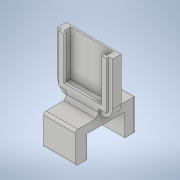
# Autodesk Inventor part: Tilt_Camera_Servo_Mount
Saved by Autodesk Inventor 2022 (Build 260153000, 153)
## iProperties
Created: 2019-12-31
Part Number: Tilt_Camera_Servo_Mount
Material: Generic
Document SubType Name: Modeling
Designer: KappaCat
Density: 1 g/cm^3
Appearance: Default
Author: KappaCat
Autodesk Inventor part; units mm, degrees
ref_plane "YZ Plane" through (0, 0, 0) normal (1, 0, 0) x (0, 1, 0)
ref_plane "XZ Plane" through (0, 0, 0) normal (0, 1, 0) x (-1, 0, 0)
ref_plane "XY Plane" through (0, 0, 0) normal (0, 0, 1) x (1, 0, 0)
sketch "Sketch1" plane through (0, 0, 0) normal (0, 1, 0) x (-1, 0, 0)
  line L0 (0, 0) -> (25.4, 0)
  line L1 (25.4, 0) -> (25.4, -50)
  line L2 (25.4, -50) -> (0, -50)
  line L3 (0, -50) -> (0, 0)
  dimension "d0" = 25.4
  dimension "d1" = 50
  constraints: 8 end point, 2 parallel, 1 horizontal, 1 perpendicular
  measures "d0" distance of L1.end L2.end
  measures "d1" distance of L0.end L1.end
extrude "Extrusion1" add sketch "Sketch1" along normal blind 5
sketch "Sketch2" plane through (0, 5, 0) normal (0, 1, 0) x (1, 0, 0)
  line L0 (-25.4, 0) -> (0, 0) projected
  line L1 (-25.4, 0) -> (0, 0)
  line L2 (0, 0) -> (0, 9.5)
  line L3 (0, 9.5) -> (-25.4, 9.5)
  line L4 (-25.4, 9.5) -> (-25.4, 0)
  line L5 (0, 0) -> (0, 50) construction
  line L6 (-25.4, 50) -> (-25.4, 0) construction
  line L7 (0, 50) -> (-25.4, 50)
  line L8 (-25.4, 50) -> (-25.4, 40.5)
  line L9 (-25.4, 40.5) -> (0, 40.5)
  line L10 (0, 40.5) -> (0, 50)
  line L11 (-18.4, 4) -> (-3.2, 4) construction
  line L12 (-3.2, 4) -> (-3.2, 46) construction
  line L13 (-3.2, 46) -> (-18.4, 46) construction
  line L14 (-18.4, 46) -> (-18.4, 4) construction
  line L15 (-10.8, 6.25) -> (-10.8, 43.75) construction
  line L16 (-3.2, 9.5) -> (-18.4, 9.5) construction
  line L17 (-18.4, 40.5) -> (-3.2, 40.5) construction
  line L18 (-12.3588, 9.5) -> (-12.3588, 40.5) construction
  line L19 (-25.4, 40.5) -> (-18.4, 40.5)
  line L20 (-18.4, 40.5) -> (-18.4, 9.5)
  line L21 (-18.4, 9.5) -> (-25.4, 9.5)
  line L22 (-25.4, 9.5) -> (-25.4, 40.5)
  point P0 (-10.8, 25)
  point P1 (-18.4, 25)
  point P2 (-10.8, 4)
  point P3 (-12.3588, 25)
  dimension "d4" = 42
  dimension "d5" = 15.2
  dimension "d6" = 37.5
  dimension "d7" = 31
  dimension "d14" = 7
  constraints: 40 end point, 8 parallel, 7 perpendicular, 7 point on line, 4 collinear, 4 horizontal, 4 midpoint, 2 horizontal alignment, 2 vertical alignment, 1 vertical
  measures "d4" distance of L13.end L11.start
  measures "d5" distance of L12.end L13.end
  measures "d6" distance of L15.end L15.start
  measures "d7" distance of L18.start L18.end
  measures "d14" distance between parallel lines of L22 L20
extrude "Extrusion2" add sketch "Sketch2" along normal blind 21
sketch "Sketch6" plane through (0, 0, 0) normal (0, -1, 0) x (1, 0, 0)
  circle A0 centre (-9.55, -18) radius 3
  line L0 (0, -50) -> (0, 0) projected
  line L1 (0, 0) -> (-25.4, 0) projected
  dimension "d24" = 6
  dimension "d25" = 9.55
  dimension "d26" = 18
  constraints: 1 centre point
  measures "d24" diameter of A0
  measures "d25" distance from line of L0 A0.centre
  measures "d26" distance from line of L1 A0.centre
extrude "Extrusion6" cut sketch "Sketch6" against normal up to next
fillet "Fillet1" radius 2 6 edges at (-25.4, 13, 0) (0, 13, 0) (-25.4, 13, -50) (-12.7, 0, -50) (-12.7, 26, -50) (0, 13, -50)
sketch "Sketch8" plane through (-25.4, 0, -48) normal (-1, 0, 0) x (0, 0, 1)
  line L0 (38.5, 26) -> (7.5, 26) projected
  line L1 (46, 0) -> (0, 0) projected
  line L2 (23, 13) -> (23, 35.5)
  line L3 (23, 13) -> (23, -9.5)
  line L4 (23, 35.5) -> (27, 35.5)
  line L5 (23, -9.5) -> (20, -9.5)
  line L6 (20, -9.5) -> (27, -9.5)
  line L7 (27, -9.5) -> (27, 35.5)
  line L8 (27, 35.5) -> (20, 35.5)
  line L9 (20, 35.5) -> (20, -9.5)
  point P0 (48, 0)
  point P1 (23, -9.5)
  point P2 (23, 35.5)
  dimension "d33" = 22.5
  dimension "d34" = 22.5
  dimension "d35" = 4
  dimension "d36" = 3
  constraints: 16 end point, 3 horizontal, 2 parallel, 1 perpendicular
  measures "d33" distance of L2.start L2.end
  measures "d34" distance of L2.start L3.end
  measures "d35" distance of L2.end L4.end
  measures "d36" distance of L3.end L5.end
extrude "Extrusion8" add sketch "Sketch8" along normal blind 45
sketch "Sketch9" plane through (-70.4, 0, -48) normal (-1, 0, 0) x (0, 0, 1)
  line L0 (27, -9.5) -> (27, 35.5) projected
  line L1 (20, 35.5) -> (20, -9.5) projected
  line L2 (23.5, 13) -> (23.5, -4.5)
  line L3 (23.5, -4.5) -> (27, -4.5)
  line L4 (23.5, 13) -> (23.5, 30.5)
  line L5 (23.5, 30.5) -> (27, 30.5)
  line L6 (27, 30.5) -> (27, -4.5)
  point P0 (48, 0)
  dimension "d39" = 17.5
  dimension "d40" = 17.5
  constraints: 10 end point, 3 point on line, 2 perpendicular, 1 collinear, 1 vertical
  measures "d39" distance of L2.start L2.end
  measures "d40" distance of L2.start L4.end
extrude "Extrusion9" cut sketch "Sketch9" against normal blind 37
sketch "Sketch10" plane through (-70.4, -4.5, -24.5) normal (0, 0, 1) x (1, 0, 0)
  line L0 (0, 0) -> (0, 35) projected
  line L1 (37, 35) -> (37, 0) projected
  line L2 (0, 0) -> (37, 0)
  line L3 (37, 0) -> (37, 35)
  line L4 (37, 35) -> (0, 35)
  line L5 (0, 35) -> (0, 0)
  point P0 (70.4, 4.5)
  constraints: 8 end point, 2 parallel, 1 horizontal, 1 perpendicular
extrude "Extrusion10" cut sketch "Sketch10" against normal blind 2
sketch "Sketch11" plane through (-25.4, -9.5, -21) normal (0, 0, 1) x (1, 0, 0)
  line L0 (-8, 5) -> (-45, 5) projected
  line L1 (-45, 5) -> (-45, 3)
  line L2 (-45, 0) -> (-45, 5) projected
  line L3 (-6, 5) -> (-6, 3)
  line L4 (-6, 3) -> (-45, 3)
  line L5 (-8, 40) -> (-8, 5) projected
  line L6 (-6, 5) -> (-6, 42)
  line L7 (-6, 42) -> (-45, 42)
  line L8 (-45, 45) -> (-45, 0) projected
  line L9 (-45, 40) -> (-8, 40) projected
  line L10 (-45, 42) -> (-45, 40)
  line L11 (-45, 40) -> (-45, 38)
  line L12 (-45, 38) -> (-10, 38)
  line L13 (-10, 38) -> (-10, 7)
  line L14 (-10, 7) -> (-45, 7)
  line L15 (-45, 5) -> (-45, 7)
  point P0 (25.4, 9.5)
  dimension "d45" = 2
  dimension "d46" = 2
  dimension "d48" = 2
  dimension "d49" = 35
  dimension "d50" = 31
  constraints: 22 end point, 4 perpendicular, 4 point on line, 2 vertical, 1 collinear, 1 horizontal
  measures "d45" distance of L0.end L1.end
  measures "d46" distance of L0.start L3.start
  measures "d48" distance of L9.start L11.end
  measures "d49" distance of L11.end L12.end
  measures "d50" distance of L12.end L13.end
extrude "Extrusion11" add sketch "Sketch11" along normal blind 2 contours L5 L9 L8 L7 L6 L3 L4 L1 L0 | L0 L8 L14 L13 L12 L9 L5
sketch "Sketch12" plane through (0, 5, 0) normal (0, 1, 0) x (1, 0, 0)
  line L0 (-18.4, 40.5) -> (-18.4, 9.5) projected
  line L1 (0, 40.5) -> (-18.4, 40.5) projected
  line L2 (-18.4, 9.5) -> (0, 9.5)
  line L3 (0, 9.5) -> (0, 40.5)
  line L4 (0, 40.5) -> (-18.4, 40.5)
  line L5 (-18.4, 40.5) -> (-18.4, 9.5)
  circle A0 centre (-9.55, 18) radius 3 projected
  circle A1 centre (-9.55, 18) radius 3
  point P0 (0, 0)
  constraints: 8 end point, 2 parallel, 1 centre point, 1 coincident, 1 horizontal, 1 perpendicular
extrude "Extrusion12" cut sketch "Sketch12" against normal blind 3
fillet "Fillet2" radius 9.5 2 edges at (-25.4, 35.5, -24.5) (-25.4, -9.5, -24.5)
sketch "Sketch13" plane through (0, 0, 0) normal (0, -1, 0) x (1, 0, 0)
  line L0 (-31.4, -21) -> (-31.4, -19) projected
  line L1 (-28.5437, -19) -> (-25.4, -16.7988)
  line L2 (-25.4, -2) -> (-25.4, -21) projected
  line L3 (-31.4, -21) -> (-24.0754, -21) construction
  line L4 (-25.4, -16.7988) -> (-25.4, -21)
  line L5 (-25.4, -21) -> (-31.4, -21)
  line L6 (-31.4, -19) -> (-70.4, -19) projected
  line L7 (-31.4, -19) -> (-28.5437, -19)
  line L8 (-25.4, -28) -> (-34.9, -28) projected
  line L9 (-31.4, -28) -> (-25.4, -32.2012)
  line L10 (-25.4, -28) -> (-25.4, -48) projected
  line L11 (-31.4, -28) -> (-24.0754, -28) construction
  line L12 (-25.4, -32.2012) -> (-25.4, -28)
  line L13 (-25.4, -28) -> (-31.4, -28)
  point P0 (0, 0)
  dimension "d56" = 35
  dimension "d57" = 35
  constraints: 18 end point, 3 collinear, 3 point on line, 2 horizontal, 2 perpendicular, 1 equal length
  measures "d56" angle of L3 L1
  measures "d57" angle of L9 L11
extrude "Extrusion13" add sketch "Sketch13" against normal up to surface (26 mm away)
sketch "Sketch14" plane through (0, 2, 0) normal (0, 1, 0) x (1, 0, 0)
  line L0 (-18.4, 9.5) -> (-18.4, 40.5) projected
  line L1 (0, 40.5) -> (0, 9.5) projected
  line L2 (-18.4, 23.418) -> (0, 23.418)
  line L3 (0, 23.418) -> (0, 30.6155)
  line L4 (0, 30.6155) -> (-18.4, 30.6155)
  line L5 (-18.4, 30.6155) -> (-18.4, 23.418)
  point P0 (0, 0)
  point P1 (0, 23.418)
  constraints: 8 end point, 2 parallel, 2 point on line, 1 horizontal, 1 perpendicular
extrude "Extrusion14" cut sketch "Sketch14" against normal through all
body "Solid1"
